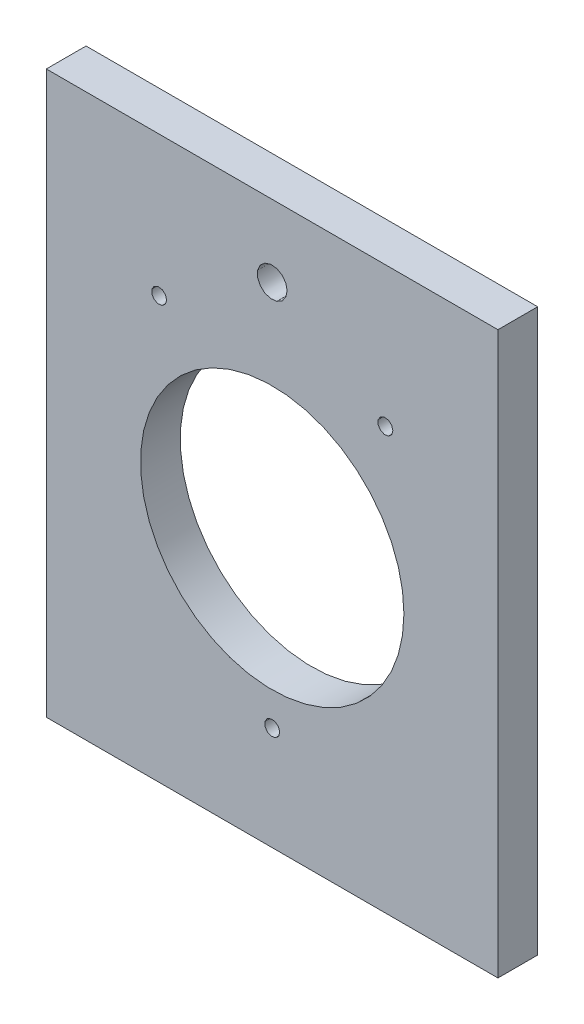
# Autodesk Inventor part: Lidar
Saved by Autodesk Inventor 2026.1 (Build 301233020, 233B)
## iProperties
Created: 2025-12-01
Part Number: Lidar
Material: 일반
Document SubType Name: Modeling
Designer: jaewook
Density: 1 g/cm^3
Appearance: 기본값
Author: jaewook
Autodesk Inventor part; units mm, degrees
ref_plane "YZ Plane" through (0, 0, 0) normal (1, 0, 0) x (0, 1, 0)
ref_plane "XZ Plane" through (0, 0, 0) normal (0, 1, 0) x (-1, 0, 0)
ref_plane "XY Plane" through (0, 0, 0) normal (0, 0, 1) x (1, 0, 0)
sketch "스케치4" plane through (0, 0, 0) normal (0, 0, 1) x (1, 0, 0)
  circle A0 centre (264.0912, 143.5876) radius 1.9
  circle A1 centre (235.6112, 63.5885) radius 1.9
  circle A2 centre (292.5662, 63.5867) radius 1.9
  circle A3 centre (264.0899, 46.4242) radius 3.75
  circle A4 centre (264.0899, 102.1242) radius 33.15
  circle A5 centre (292.5662, 63.5867) radius 1.5
  circle A6 centre (235.6112, 63.5885) radius 1.5
  circle A7 centre (264.0912, 143.5876) radius 1.5
  line L0 (264.0899, 102.1242) -> (264.0899, 46.4242)
  line L1 (356.232, 0) -> (158.7026, 0)
  circle A8 centre (264.0912, -143.5876) radius 1.9
  circle A9 centre (235.6112, -63.5885) radius 1.9
  circle A10 centre (292.5662, -63.5867) radius 1.9
  circle A11 centre (264.0899, -46.4242) radius 3.75
  circle A12 centre (264.0899, -102.1242) radius 33.15
  circle A13 centre (235.6112, -63.5885) radius 1.5
  circle A14 centre (264.0912, -143.5876) radius 1.5
  circle A15 centre (292.5662, -63.5867) radius 1.5
  line L2 (264.0899, -102.1242) -> (264.0899, -46.4242) construction
  line L3 (320.9052, -28.3469) -> (207.2359, -28.3469)
  line L4 (207.2359, -28.3469) -> (207.2359, -169.6626)
  line L5 (207.2359, -169.6626) -> (320.9052, -169.6626)
  line L6 (320.9052, -169.6626) -> (320.9052, -28.3469)
  point P0 (0, 0)
  dimension "d38" = 3
  dimension "d39" = 3
  dimension "d40" = 3
  dimension "d41" = 41.4634
  dimension "d42" = 47.917
  dimension "d45" = 7.5
  dimension "d48" = 143.537
  dimension "d50" = 47.917
  dimension "d51" = 36.465
  dimension "d52" = 36.462
  dimension "d53" = 179.998
  dimension "d54" = 55.7
  constraints: 16 centre point, 14 end point, 8 symmetric about line, 6 coincident, 2 horizontal, 2 parallel, 1 perpendicular, 1 vertical, 8 other
  measures "d38" diameter of A5
  measures "d39" diameter of A6
  measures "d40" diameter of A7
  measures "d41" distance of L0.start A0.centre
  measures "d42" distance of A1.centre L0.start
  measures "d45" diameter of A3
  measures "d50" distance of L0.start A2.centre
  measures "d54" distance of L0.end L0.start
extrude "돌출3" add sketch "스케치4" along normal blind 10 contours L6 L5 L4 L3
